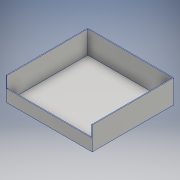
# Autodesk Inventor part: BatteryHolder-ver1-1111-2019
Saved by Autodesk Inventor 2018 (Build 220112000, 112)
## iProperties
Created: 2019-12-12
Part Number: BatteryHolder-ver1-1111-2019
Material: Aluminum 6061
Document SubType Name: Modeling
Designer: JMHal
Density: 2.7 g/cm^3
Appearance: Aluminum - Flat
Author: JMHal
Autodesk Inventor part; units mm, degrees
ref_plane "YZ Plane" through (0, 0, 0) normal (1, 0, 0) x (0, 1, 0)
ref_plane "XZ Plane" through (0, 0, 0) normal (0, 1, 0) x (-1, 0, 0)
ref_plane "XY Plane" through (0, 0, 0) normal (0, 0, 1) x (1, 0, 0)
sketch "Sketch1" plane through (0, 0, 0) normal (0, 0, 1) x (1, 0, 0)
  line L0 (0, 0) -> (187.325, 0)
  line L1 (187.325, 0) -> (187.325, 177.8)
  line L2 (187.325, 177.8) -> (0, 177.8)
  line L3 (0, 177.8) -> (0, 0)
  dimension "d0" = 177.8
  dimension "d1" = 187.325
  constraints: 8 end point, 2 parallel, 1 horizontal, 1 perpendicular
  measures "d0" distance of L0.end L1.end
  measures "d1" distance of L1.end L2.end
extrude "Extrusion1" add sketch "Sketch1" along normal blind 50.8
shell "Shell1" thickness 1.5875 removed faces 1 at (124.8833, 59.2667, 50.8)
sketch "Sketch2" plane through (0, 0, 0) normal (0, -1, 0) x (1, 0, 0)
  line L0 (185.7375, 1.5875) -> (185.7375, 50.8) projected
  line L1 (1.5875, 50.8) -> (185.7375, 50.8)
  line L2 (185.7375, 50.8) -> (185.7375, 26.1937)
  line L3 (185.7375, 26.1937) -> (1.5875, 26.1937)
  line L4 (1.5875, 26.1937) -> (1.5875, 50.8)
  line L5 (1.5875, 1.5875) -> (1.5875, 50.8) projected
  line L6 (0, 50.8) -> (187.325, 50.8) projected
  point P0 (0, 0)
  point P1 (1.5875, 26.1937)
  point P2 (93.6625, 50.8)
  constraints: 8 end point, 3 midpoint, 2 parallel, 1 coincident, 1 horizontal, 1 horizontal alignment, 1 perpendicular
extrude "Extrusion2" cut sketch "Sketch2" against normal up to surface (1.5875 mm away)
body "Solid1"
